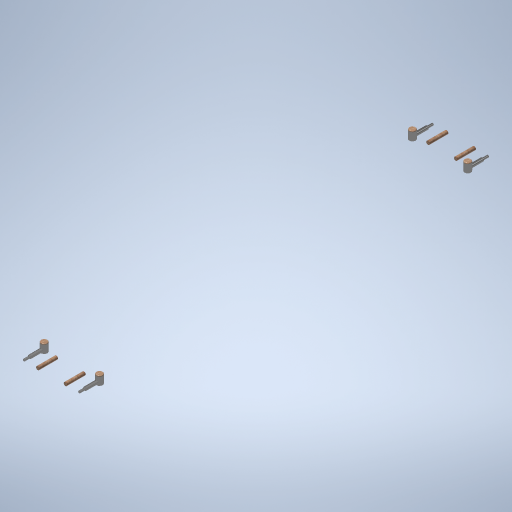
# Autodesk Inventor part: REC_05
Saved by Autodesk Inventor 2024.3 (Build 283343000, 343)
## iProperties
RuleStatus: InUse
Created: 2014-05-08
Part Number: REC_05
Material: Generic
Document SubType Name: Modeling
Designer: SauliusD
Density: 1 g/cm^3
Appearance: Default
Description: Pillar Board & 2 Nestled Boards from Sides Minifixes-05
AfterDocNew0: Fire Form
Author: SauliusD
Autodesk Inventor part; units mm, degrees
sketch "Sketch2" plane through (0, 0, 0) normal (0, 0, 1) x (1, 0, 0)
  line L0 (277.7589, -758.1253) -> (141.7589, -758.1253)
  line L1 (141.7589, -758.1253) -> (141.7589, 161.8747)
  line L2 (141.7589, 161.8747) -> (277.7589, 161.8747)
  line L3 (277.7589, 161.8747) -> (277.7589, -758.1253)
  point P0 (209.7589, 161.8747)
  point P1 (141.7589, -298.1253)
  constraints: 8 end point, 2 midpoint, 2 parallel, 1 horizontal, 1 perpendicular
ref_plane "Work Plane1" through (0, 0, -12.5) normal (0, 0, 1) x (1, 0, 0)
sketch "Sketch3" plane through (0, 0, -12.5) normal (0, 0, 1) x (1, 0, 0)
  line L0 (277.7589, 161.8747) -> (277.7589, -758.1253) construction
  line L1 (141.7589, 161.8747) -> (277.7589, 161.8747) construction
  line L2 (141.7589, -758.1253) -> (141.7589, 161.8747) construction
  line L3 (145.7589, 161.8747) -> (149.7589, 161.8747)
  line L4 (149.7589, 161.8747) -> (149.7589, 127.8747)
  line L5 (149.7589, 127.8747) -> (145.7589, 127.8747)
  line L6 (145.7589, 127.8747) -> (145.7589, 161.8747)
  line L7 (145.7589, 161.8747) -> (148.2589, 161.8747)
  line L8 (148.2589, 161.8747) -> (148.2589, 174.8747)
  line L9 (148.2589, 174.8747) -> (145.7589, 174.8747)
  line L10 (145.7589, 174.8747) -> (145.7589, 161.8747)
  line L11 (209.7589, 161.8747) -> (209.7589, 132.7708) construction
  line L12 (273.7589, 127.8747) -> (273.7589, 161.8747)
  point P0 (0, 0)
  dimension "d5" = 8
  dimension "d7" = 5
  dimension "d8" = 13
  dimension "Dist_Between_Planes" = 136
  dimension "Distance_between_Axis" = 128
  constraints: 20 end point, 5 parallel, 2 horizontal, 2 perpendicular, 2 symmetric about line, 1 collinear, 1 midpoint, 1 vertical alignment
  measures "d5" diameter of L4 L6
  measures "d7" diameter of L8 L10
  measures "d8" distance of L7.end L8.end
  measures "Dist_Between_Planes" distance of L1.start L0.start
  measures "Distance_between_Axis" distance between parallel lines of L6 L12
revolve "Minifix Revolve" add sketch "Sketch3" angle 360 about axis through (145.7589, 174.8747, -12.5) along (0, -1, 0)
sketch "Sketch4" plane through (0, 0, -12.5) normal (0, 0, 1) x (1, 0, 0)
  line L0 (141.7589, 127.8747) -> (149.7589, 127.8747) construction
  circle A0 centre (145.7589, 127.8747) radius 7.5
  point P0 (0, 0)
  dimension "d10" = 15
  constraints: 1 centre point, 1 midpoint
  measures "d10" diameter of A0
extrude "Minifix Extrude" add sketch "Sketch4" along normal up to surface (12.5 mm away)
extrude "Minifix extrude 2" add sketch "Sketch4" against normal blind 6
ref_plane "Work Plane2" through (209.7589, 161.8747, 0) normal (1, 0, 0) x (0, 1, 0)
ref_plane "Work Plane3" through (141.7589, -298.1253, 0) normal (0, 1, 0) x (-1, 0, 0)
sketch "Sketch5" plane through (0, 0, -12.5) normal (0, 0, 1) x (1, 0, 0)
  line L0 (145.7589, 361.4747) -> (145.7589, -944.7253) construction
  line L1 (177.7589, 174.8747) -> (177.7589, 131.8747)
  line L2 (177.7589, 174.8747) -> (181.7589, 174.8747)
  line L3 (181.7589, 174.8747) -> (181.7589, 131.8747)
  line L4 (181.7589, 131.8747) -> (177.7589, 131.8747)
  line L5 (143.2589, 174.8747) -> (148.2589, 174.8747) construction
  line L6 (141.7589, 161.8747) -> (149.7589, 161.8747) construction
  point P0 (0, 0)
  dimension "Dowel_D" = 8
  dimension "Dowel_Drill_Depth" = 30
  dimension "d17" = 32
  constraints: 8 end point, 2 parallel, 2 perpendicular, 1 collinear
  measures "Dowel_D" diameter of L3 L1
  measures "Dowel_Drill_Depth" distance between parallel lines of L4 L6
  measures "d17" distance from line of L1.start L0
revolve "Dowel Revolve" add sketch "Sketch5" angle 360 about axis through (177.7589, 174.8747, -12.5) along (0, -1, 0) separate body
mirror "Mirror1" about plane through (209.7589, 161.8747, 0) normal (1, 0, 0) of "Minifix Extrude", "Minifix Revolve", "Dowel Revolve", "Minifix extrude 2" bodies 1
sketch "Sketch6" plane through (0, 0, -12.5) normal (0, 0, 1) x (1, 0, 0)
  point P0 (0, 0)
sketch "Sketch7" plane through (0, 0, -12.5) normal (0, 0, 1) x (1, 0, 0)
  line L0 (209.7589, 361.4747) -> (209.7589, -944.7253) construction
  line L1 (212.2589, 161.8747) -> (209.7589, 161.8747)
  line L2 (209.7589, 161.8747) -> (209.7589, 174.8747)
  line L3 (209.7589, 174.8747) -> (212.2589, 174.8747)
  line L4 (212.2589, 174.8747) -> (212.2589, 161.8747)
  line L5 (209.7589, 161.8747) -> (213.7589, 161.8747)
  line L6 (213.7589, 161.8747) -> (213.7589, 127.8747)
  line L7 (213.7589, 127.8747) -> (209.7589, 127.8747)
  line L8 (209.7589, 127.8747) -> (209.7589, 161.8747)
  line L9 (143.2589, 174.8747) -> (148.2589, 174.8747) construction
  line L10 (141.7589, 161.8747) -> (149.7589, 161.8747) construction
  point P0 (0, 0)
  point P1 (209.7589, -944.7253)
  dimension "d19" = 34
  dimension "d20" = 5
  dimension "d21" = 8
  constraints: 16 end point, 4 parallel, 2 collinear, 2 horizontal, 2 perpendicular, 1 vertical, 1 other
  measures "d19" distance of L5.end L6.end
  measures "d20" diameter of L4 L2
  measures "d21" diameter of L6 L2
revolve "Center minixix Revolution" [suppressed]
sketch "Sketch8" plane through (0, 0, -12.5) normal (0, 0, 1) x (1, 0, 0)
  circle A0 centre (209.7589, 127.8747) radius 7.5
  line L0 (213.7589, 127.8747) -> (209.7589, 127.8747) construction
  point P0 (0, 0)
  dimension "d23" = 15
  constraints: 1 centre point, 1 coincident
  measures "d23" diameter of A0
extrude "Center minixix Extrusion 1" [suppressed]
extrude "Center minixix Extrusion 2" [suppressed]
ref_plane "Work Plane4" through (277.7589, 161.8747, 0) normal (0, 1, 0) x (-1, 0, 0)
mirror "Mirror2" about plane through (141.7589, -298.1253, 0) normal (0, 1, 0) of "Minifix Extrude", "Minifix Revolve", "Dowel Revolve", "Minifix extrude 2", "Mirror1" bodies 1
mirror "Mirror Center" [suppressed]
sketch "Sketch9" plane through (145.7589, 127.8747, 0) normal (0, 0, 1) x (1, 0, 0)
  circle A0 centre (0, 0) radius 7.5 projected
  point P0 (-145.7589, -127.8747)
extrude "Side Cover Cap Extrusion" add sketch "Sketch9" along normal blind 2 separate body
fillet "Side Cover Cap Fillet" radius 1.6 1 edges at (138.2589, 127.8747, 2)
mirror "Mirror3" about plane through (209.7589, 161.8747, 0) normal (1, 0, 0) of "Side Cover Cap Extrusion", "Side Cover Cap Fillet" bodies 3
mirror "Mirror4" about plane through (141.7589, -298.1253, 0) normal (0, 1, 0) of "Side Cover Cap Extrusion", "Side Cover Cap Fillet", "Mirror3" bodies 3
sketch "Sketch10" plane through (0, 0, 0) normal (0, 0, 1) x (1, 0, 0)
  circle A0 centre (209.7589, 127.8747) radius 7.5
  line L0 (141.7589, 161.8747) -> (277.7589, 161.8747) projected
  point P0 (18.2411, -127.8747)
  point P1 (209.7589, 161.8747)
  dimension "d42" = 34
  constraints: 1 centre point, 1 midpoint, 1 vertical alignment
  measures "d42" distance from line of L0 A0.centre
extrude "Center Cover Cap Extrusion" [suppressed]
fillet "Center Cover Cap Fillet" [suppressed]
mirror "Mirror5" [suppressed]
revolve "Center Dowel Revolve" [suppressed]
mirror "Mirror7" [suppressed]
mirror "Mirror8" [suppressed]
sketch "Sketch11" plane through (0, 0, -12.5) normal (0, 0, 1) x (1, 0, 0)
  line L0 (209.7589, 348.4747) -> (209.7589, -957.7253) construction
  line L1 (173.7589, -771.1253) -> (177.7589, -771.1253)
  line L2 (177.7589, -771.1253) -> (177.7589, -728.1253)
  line L3 (177.7589, -728.1253) -> (173.7589, -728.1253)
  line L4 (173.7589, -728.1253) -> (173.7589, -771.1253)
  line L5 (245.7589, -771.1253) -> (237.7589, -771.1253) construction
  line L6 (245.7589, -728.1253) -> (237.7589, -728.1253) construction
  point P0 (0, 0)
  dimension "d43" = 8
  dimension "d44" = 32
  constraints: 8 end point, 2 collinear, 2 parallel, 1 horizontal, 1 perpendicular
  measures "d43" diameter of L4 L2
  measures "d44" distance from line of L1.end L0
equation "\"d23\" = d10"
equation "\"d38\" = d35"
equation "\"d20\" = d7"
equation "\"d21\" = d5"
equation "\"d43\" = Dowel_D"
equation "\"d44\" = Step"
equation "\"Step\" = 32"
equation "\"d35\" = 1.6"
